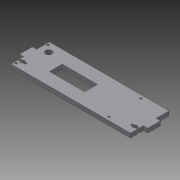
# Autodesk Inventor part: Controller_Front
Saved by Autodesk Inventor 2014 (Build 180170000, 170)
## iProperties
Created: 2014-11-10
Part Number: Controller_Front
Material: Generic
Document SubType Name: Modeling
Designer: ThatOtherGuy
Density: 1 g/cm^3
Appearance: Default
Author: ThatOtherGuy
Autodesk Inventor part; units mm, degrees
ref_plane "YZ Plane" through (0, 0, 0) normal (1, 0, 0) x (0, 1, 0)
ref_plane "XZ Plane" through (0, 0, 0) normal (0, 1, 0) x (-1, 0, 0)
ref_plane "XY Plane" through (0, 0, 0) normal (0, 0, 1) x (1, 0, 0)
sketch "Sketch1" plane through (0, 0, 0) normal (0, 0, 1) x (1, 0, 0)
  line L0 (0, 0) -> (186.538, 0)
  line L1 (186.538, 0) -> (186.538, 60)
  line L2 (186.538, 60) -> (0, 60)
  line L3 (0, 60) -> (0, 0)
  dimension "d0" = 186.538
  dimension "d1" = 60
  constraints: 8 end point, 2 parallel, 1 horizontal, 1 perpendicular
  measures "d0" distance of L1.end L2.end
  measures "d1" distance of L2.end L0.start
extrude "Extrusion1" add sketch "Sketch1" along normal blind 6.731
sketch "Sketch2" plane through (0, 0, 6.731) normal (0, 0, 1) x (1, 0, 0)
  line L0 (186.538, 0) -> (186.538, 60) projected
  line L1 (0, 60) -> (0, 0) projected
  line L2 (186.538, 40) -> (193.269, 40)
  line L3 (193.269, 40) -> (193.269, 20)
  line L4 (193.269, 20) -> (186.538, 20)
  line L5 (186.538, 20) -> (186.538, 40)
  line L6 (0, 40) -> (-6.731, 40)
  line L7 (-6.731, 40) -> (-6.731, 20)
  line L8 (-6.731, 20) -> (0, 20)
  line L9 (0, 20) -> (0, 40)
  point P0 (0, 30)
  point P1 (0, 30)
  dimension "d4" = 20
  dimension "d5" = 6.731
  constraints: 16 end point, 4 parallel, 2 equal length, 2 horizontal, 2 midpoint, 2 perpendicular, 2 point on line, 1 coincident, 1 collinear
  measures "d4" distance of L6.end L7.end
  measures "d5" distance of L6.start L6.end
extrude "Tabs" add sketch "Sketch2" against normal blind 6.731
sketch "Sketch5" plane through (0, 0, 6.731) normal (0, 0, 1) x (1, 0, 0)
  line L0 (193.269, 40) -> (186.538, 40) projected
  line L1 (0, 40) -> (-6.731, 40) projected
  line L2 (-6.731, 40) -> (-6.731, 20) projected
  point P0 (-3.3655, 30)
  point P1 (189.9035, 30)
  point P2 (-6.731, 30)
  point P3 (-6.731, 30)
  point P4 (189.9035, 40)
  point P5 (-3.3655, 40)
  constraints: 4 midpoint, 2 horizontal alignment, 2 vertical alignment
hole "TabHole" [suppressed]
sketch "Sketch3" plane through (0, 0, 6.731) normal (0, 0, 1) x (1, 0, 0)
  line L0 (0, 60) -> (0, 40) projected
  line L1 (-6.731, 40) -> (-6.731, 20) projected
  line L2 (40, 40) -> (95, 40)
  line L3 (95, 40) -> (95, 20)
  line L4 (95, 20) -> (40, 20)
  line L5 (40, 20) -> (40, 40)
  point P0 (40, 30)
  point P1 (-6.731, 30)
  dimension "d8" = 55
  dimension "d9" = 20
  dimension "d10" = 40
  constraints: 8 end point, 2 midpoint, 2 parallel, 1 horizontal, 1 horizontal alignment, 1 perpendicular
  measures "d8" distance of L2.start L2.end
  measures "d9" distance of L4.end L2.start
  measures "d10" distance between parallel lines of L0 L5
extrude "RibbonHole" cut sketch "Sketch3" against normal up to next
sketch "Sketch4" plane through (0, 0, 6.731) normal (0, 0, 1) x (1, 0, 0)
  line L0 (40, 20) -> (40, 40) projected
  line L1 (0, 60) -> (0, 40) projected
  line L2 (0, 20) -> (0, 0) projected
  line L3 (3, 5.235) -> (3, 54.765) construction
  line L4 (3, 54.765) -> (147.78, 54.765) construction
  point P0 (3, 30)
  point P1 (40, 30)
  point P2 (147.78, 5.235)
  dimension "d13" = 144.78
  dimension "d14" = 49.53
  dimension "d16" = 3
  constraints: 4 end point, 3 coincident, 2 horizontal alignment, 2 midpoint, 1 parallel, 1 perpendicular, 1 vertical alignment
  measures "d13" distance of L3.end L4.end
  measures "d14" distance of L3.start L3.end
  measures "d16" distance between parallel lines of L1 L3
hole "LCDMount" at (3, 54.765, 6.731) at (147.78, 54.765, 6.731) at (147.78, 5.235, 6.731) at (3, 5.235, 6.731) direction (0, 0, -1) diameter 3.176 end through all
sketch "Sketch6" plane through (0, 0, 6.731) normal (0, 0, 1) x (1, 0, 0)
  line L0 (186.538, 60) -> (0, 60) projected
  line L1 (0, 60) -> (0, 40) projected
  circle A0 centre (13.5, 45.5) radius 5
  dimension "d31" = 14.5
  dimension "d32" = 13.5
  dimension "d33" = 10
  constraints: 1 centre point
  measures "d31" distance from line of L0 A0.centre
  measures "d32" distance from line of L1 A0.centre
  measures "d33" diameter of A0
extrude "PotHole" cut sketch "Sketch6" against normal up to next
sketch "Sketch7" plane through (0, 0, 6.731) normal (0, 0, 1) x (1, 0, 0)
  line L0 (-6.731, 20) -> (0, 20) projected
  line L1 (0, 20) -> (0, 0) projected
  line L2 (0, 14.088) -> (4.093, 14.088)
  line L3 (4.093, 14.088) -> (4.093, 15.5)
  line L4 (4.093, 15.5) -> (7.269, 15.5)
  line L5 (7.269, 15.5) -> (7.269, 14.088)
  line L6 (7.269, 14.088) -> (11.269, 14.088)
  line L7 (11.269, 14.088) -> (11.269, 10.912)
  line L8 (11.269, 10.912) -> (7.269, 10.912)
  line L9 (7.269, 10.912) -> (7.269, 9.5)
  line L10 (7.269, 9.5) -> (4.093, 9.5)
  line L11 (4.093, 9.5) -> (4.093, 10.912)
  line L12 (4.093, 10.912) -> (0, 10.912)
  line L13 (186.538, 0) -> (186.538, 20) projected
  line L14 (-6.731, 40) -> (-6.731, 20) projected
  line L15 (186.538, 14.088) -> (182.445, 14.088)
  line L16 (182.445, 14.088) -> (182.445, 15.5)
  line L17 (182.445, 15.5) -> (179.269, 15.5)
  line L18 (179.269, 15.5) -> (179.269, 14.088)
  line L19 (179.269, 14.088) -> (175.269, 14.088)
  line L20 (175.269, 14.088) -> (175.269, 10.912)
  line L21 (175.269, 10.912) -> (179.269, 10.912)
  line L22 (179.269, 10.912) -> (179.269, 9.5)
  line L23 (179.269, 9.5) -> (182.445, 9.5)
  line L24 (182.445, 9.5) -> (182.445, 10.912)
  line L25 (182.445, 10.912) -> (186.538, 10.912)
  point P0 (11.269, 12.5)
  dimension "d36" = 3.176
  dimension "d38" = 11.269
  dimension "d39" = 4
  dimension "d40" = 6
  dimension "d43" = 7.5
  constraints: 44 end point, 16 equal length, 13 parallel, 5 collinear, 5 perpendicular, 4 point on line, 1 midpoint
  measures "d36" distance of L3.end L4.end
  measures "d38" distance between parallel lines of L1 L7
  measures "d39" distance of L5.end L6.end
  measures "d40" distance between parallel lines of L10 L4
  measures "d43" distance from line of L0 point (11.269, 12.5)
extrude "Nut" cut sketch "Sketch7" against normal up to next
equation "\"d2\" = THICKB"
equation "\"d5\" = THICKB"
equation "\"d6\" = THICKB"
equation "\"THICKA\" = 3.175"
equation "\"THICKB\" = 6.731"
equation "\"THICKC\" = 12.7"
equation "\"THICKPLY\" = 5"
equation "\"MAGDIA\" = 9.5"
equation "\"BALLDIA\" = 12"
body "Solid1"
